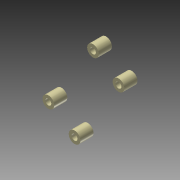
# Autodesk Inventor part: Spacer
Saved by Autodesk Inventor 2015 (Build 190159000, 159)
## iProperties
Created: 2015-01-24
Part Number: Spacer
Material: Nylon 6/6
Document SubType Name: Modeling
Designer: Brian
Density: 1.13 g/cm^3
Appearance: Nylon 6
Author: Brian
Autodesk Inventor part; units mm, degrees
ref_plane "YZ Plane" through (0, 0, 0) normal (1, 0, 0) x (0, 1, 0)
ref_plane "XZ Plane" through (0, 0, 0) normal (0, 1, 0) x (-1, 0, 0)
ref_plane "XY Plane" through (0, 0, 0) normal (0, 0, 1) x (1, 0, 0)
sketch "Sketch1" plane through (0, 0, 0) normal (0, 0, 1) x (1, 0, 0)
  circle A0 centre (-12.1068, -49.2285) radius 3.302 construction
  circle A1 centre (-40.5845, -30.3795) radius 3.302 construction
  circle A2 centre (7.8606, 42.0186) radius 3.302 construction
  circle A3 centre (35.6069, 23.6537) radius 3.302 construction
  circle A4 centre (-12.1068, -49.2285) radius 6.35
  circle A5 centre (-12.1068, -49.2285) radius 3.2004
  circle A6 centre (-40.5845, -30.3795) radius 3.2004
  circle A7 centre (-40.5845, -30.3795) radius 6.35
  circle A8 centre (35.6069, 23.6537) radius 3.2004
  circle A9 centre (35.6069, 23.6537) radius 6.35
  circle A10 centre (7.8606, 42.0186) radius 3.2004
  circle A11 centre (7.8606, 42.0186) radius 6.35
  point P0 (0, 0)
  dimension "d2" = 12.7
  dimension "d3" = 6.4008
  dimension "d4" = 6.4008
  dimension "d5" = 12.7
  dimension "d6" = 6.4008
  dimension "d7" = 12.7
  dimension "d8" = 6.4008
  dimension "d9" = 12.7
  constraints: 8 centre point, 8 coincident
  measures "d2" diameter of A4
  measures "d3" diameter of A5
  measures "d4" diameter of A6
  measures "d5" diameter of A7
  measures "d6" diameter of A8
  measures "d7" diameter of A9
  measures "d8" diameter of A10
  measures "d9" diameter of A11
extrude "Extrusion1" add sketch "Sketch1" along normal blind 14.2875
body "Solid1"
